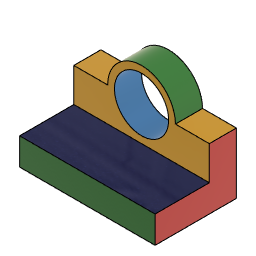
darshan_nair_exercise3 (Autodesk Fusion 360 design; units mm, degrees)
Autodesk Fusion 360 part; units mm, degrees
note: some values were not read from the file. Set by a fixed rule: which sketch regions a step uses.
sketch "Sketch1" plane through (0, 0, 0) normal (0, 0, 1) x (1, 0, 0)
  line L0 (0, 0) -> (0, 40)
  line L1 (0, 40) -> (0, 60)
  line L2 (0, 60) -> (25, 60)
  line L3 (25, 60) -> (75, 60)
  line L4 (75, 60) -> (100, 60)
  line L5 (100, 60) -> (100, 40)
  line L6 (100, 40) -> (0, 40)
  line L7 (100, 40) -> (100, 0)
  line L8 (25, 60) -> (25, 40)
  line L9 (75, 60) -> (75, 40)
  line L10 (0, 0) -> (100, 0)
  dimension "d1" = 40
  dimension "d2" = 20
  dimension "d3" = 25
  dimension "d4" = 50
  dimension "d5" = 25
  dimension "d6" = 20
  dimension "d7" = 100
  dimension "d8" = 60
  constraint coincident L0.start L10.start
  constraint vertical L0
  constraint vertical L1
  constraint perpendicular L1 L2
  constraint parallel L2 L3
  constraint parallel L3 L4
  constraint perpendicular L4 L5
  constraint perpendicular L6 L7
  constraint coincident L6 L8.end
  constraint perpendicular L6 L8
  constraint coincident L6 L9.end
  constraint perpendicular L6 L9
  constraint perpendicular L7 L10
  measures "d1" distance of L0.start L0.end
  measures "d2" distance of L0.end L1.end
  measures "d3" distance of L1.end L2.end
  measures "d4" distance of L2.end L3.end
  measures "d5" distance of L3.end L4.end
  measures "d6" distance of L4.end L5.end
  measures "d7" distance of L0.start L7.end
  measures "d8" distance of L4.end L7.end
extrude "Extrude1" add sketch "Sketch1" along normal blind 20 contours L0 L6 L7 L10
extrude "Extrude2" add sketch "Sketch1" along normal blind 45 contours L1 L2 L6 L8 | L3 L6 L8 L9 | L4 L5 L6 L9
sketch "Sketch2" plane through (0, 40, 0) normal (0, -1, 0) x (1, 0, 0)
  line L0 (0, 20) -> (100, 20)
  line L1 (100, 20) -> (100, 45)
  line L2 (100, 45) -> (0, 45)
  line L3 (0, 45) -> (0, 20)
  circle A0 centre (50, 45) radius 20
  circle A1 centre (50, 45) radius 25
  dimension "d13" = 40
  dimension "d14" = 50
  constraint midpoint L2 A0.centre
  constraint concentric A0 A1
  measures "d13" diameter of A0
  measures "d14" diameter of A1
extrude "Extrude4" cut sketch "Sketch2" against normal blind 105 contours L2 A0 picked at (49.5018, 38.352)
extrude "Extrude3" add sketch "Sketch2" against normal blind 20 contours L2 A0 A1 picked at (26.7597, 46.242)
sketch "Sketch3" plane through (0, 40, 0) normal (0, -1, 0) x (1, 0, 0)
  line L0 (25, 45) -> (0, 45)
  line L1 (0, 45) -> (0, 20)
  line L2 (0, 20) -> (100, 20)
  line L3 (100, 20) -> (100, 45)
  line L4 (100, 45) -> (75, 45)
  arc A0 (75, 45) -> (25, 45) centre (50, 45) ccw
  circle A1 centre (50, 45) radius 20
  point P0 (100, 20)
  point P1 (100, 0)
  dimension "d17" = 100
  dimension "d18" = 20
  dimension "d19" = 50
  measures "d17" distance of L1.end P0
  measures "d18" distance of P0 P1
  measures "d19" distance of L0.end A0.centre
sketch "Sketch4" plane through (100, 0, 0) normal (1, 0, 0) x (0, 1, 0)
  line L0 (0, 0) -> (60, 0)
  line L1 (60, 0) -> (60, 45)
  line L2 (60, 45) -> (40, 45)
  line L3 (40, 45) -> (40, 20)
  line L4 (40, 20) -> (0, 20)
  line L5 (0, 20) -> (0, 0)
  line L6 (60, 0, -25) -> (60, 0, 0)
  point P0 (60, 0)
  dimension "d20" = 45
  dimension "d21" = 60
  measures "d20" distance of L1.end P0
